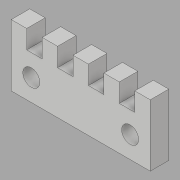
# Autodesk Inventor part: e_rail support
Saved by Autodesk Inventor 2019 (Build 230136000, 136)
## iProperties
Created: 2021-11-03
Part Number: e_rail support
Material: Generic
Document SubType Name: Modeling
Designer: Mohamed
Density: 1 g/cm^3
Appearance: Default
Author: Mohamed
Autodesk Inventor part; units mm, degrees
ref_plane "YZ Plane" through (0, 0, 0) normal (1, 0, 0) x (0, 1, 0)
ref_plane "XZ Plane" through (0, 0, 0) normal (0, 1, 0) x (-1, 0, 0)
ref_plane "XY Plane" through (0, 0, 0) normal (0, 0, 1) x (1, 0, 0)
sketch "Sketch1" plane through (0, 0, 0) normal (0, 0, 1) x (1, 0, 0)
  line L0 (0, 0) -> (45, 0)
  line L1 (45, 0) -> (45, 20)
  line L2 (45, 20) -> (0, 20)
  line L3 (0, 20) -> (0, 0)
  circle A0 centre (6.5, 7) radius 2.75
  circle A1 centre (38.5, 7) radius 2.75
  dimension "d0" = 45
  dimension "d1" = 20
  dimension "d5" = 5.5
  dimension "d6" = 5.5
  constraints: 8 end point, 2 centre point, 2 parallel, 1 horizontal, 1 perpendicular
  measures "d0" distance of L2.end L1.end
  measures "d1" distance of L1.end L0.end
  measures "d5" diameter of A0
  measures "d6" diameter of A1
extrude "Extrusion1" add sketch "Sketch1" along normal blind 6
sketch "Sketch2" plane through (0, 0, 6) normal (0, 0, 1) x (1, 0, 0)
  line L0 (45, 20) -> (0, 20) projected
  line L1 (0, 20) -> (5, 20)
  line L2 (5, 20) -> (10, 20)
  line L3 (10, 20) -> (10, 14)
  line L4 (10, 14) -> (5, 14)
  line L5 (5, 14) -> (5, 20)
  point P0 (0, 0)
  dimension "d9" = 5
  dimension "d10" = 5
  dimension "d11" = 6
  constraints: 10 end point, 2 parallel, 1 horizontal, 1 perpendicular, 1 point on line
  measures "d9" distance of L0.end L1.end
  measures "d10" distance of L3.end L4.end
  measures "d11" distance of L2.end L3.end
extrude "Extrusion2" cut sketch "Sketch2" against normal blind 6
pattern_linear "Rectangular Pattern1" count 4 spacing 10 along (1, 0, 0) of "Extrusion2"
body "Solid1"
